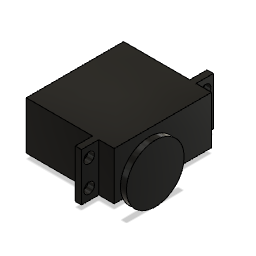
Servo Module v45 (Autodesk Fusion 360 archive; units mm, degrees)
design "HS-311"
Autodesk Fusion 360 part; units mm, degrees
sketch "Sketch1" plane through (0, 0, 0) normal (0, 0, 1) x (1, 0, 0) in component "MG995 v1 (1)"
  line L0 (-20.2, 9.95) -> (20.2, 9.95)
  line L1 (20.2, 9.95) -> (20.2, -9.95)
  line L2 (20.2, -9.95) -> (-20.2, -9.95)
  line L3 (-20.2, -9.95) -> (-20.2, 9.95)
  line L4 (0, 9.95) -> (0, -9.95) construction
  line L5 (-20.2, 0) -> (20.2, 0) construction
  dimension "d1_1_1_1_1" = 40.4
  dimension "d2_1_1_1_1" = 19.9
  constraint horizontal L0
  constraint vertical L1
  constraint horizontal L2
  constraint vertical L3
  constraint midpoint L0 L4.start
  constraint midpoint L2 L4.end
  constraint midpoint L3 L5.start
  constraint midpoint L1 L5.end
  constraint coincident origin L5
  constraint coincident origin L4
  measures "d1_1_1_1_1" distance of L0.start L0.end
  measures "d2_1_1_1_1" distance of L0.start L2.end
extrude "Extrude1" add sketch "Sketch1" along normal blind 36.5 in component "MG995 v1 (1)"
sketch "Sketch2" plane through (0, 0, 36.5) normal (0, 0, 1) x (1, 0, 0) in component "MG995 v1 (1)"
  line L0 (-20.2, -9.95) -> (20.2, -9.95)
  line L1 (20.2, -9.95) -> (20.2, 9.95)
  line L2 (20.2, 9.95) -> (-20.2, 9.95)
  line L3 (-20.2, 9.95) -> (-20.2, -9.95)
  line L4 (20.2, 9.95) -> (-20.2, 9.95)
  line L5 (-20.2, -9.95) -> (20.2, -9.95)
  line L6 (-10.7, 9.95) -> (-10.7, -9.95) construction
  circle A0 centre (-10.7, 0) radius 2.9
  line L7 (0, 9.95) -> (0, -9.95) construction
  dimension "d5_1_1_1_1" = 5.8
  dimension "d8_1_1_1_1" = 9.5
  constraint coincident L2 L6.start
  constraint coincident L0 L6.end
  constraint perpendicular L0 L6
  constraint midpoint L6 A0.centre
  constraint midpoint L4 L7.start
  constraint midpoint L5 L7.end
  measures "d5_1_1_1_1" diameter of A0
  measures "d8_1_1_1_1" distance of L3 L6
extrude "Extrude2" add sketch "Sketch2" along normal blind 5.06 contours A0 in component "MG995 v1 (1)"
ref_plane "WorkPlane1" through (0, 0, 27.5) normal (0, 0, -1) x (-1, 0, 0) in component "MG995 v1 (1)"
sketch "Sketch3" plane through (-4.1411, 18.8966, 27.5) normal (0, 0, -1) x (1, 0, 0) in component "MG995 v1 (1)"
  line L0 (31.5411, 8.9466) -> (-23.2589, 8.9466)
  line L1 (-23.2589, 8.9466) -> (-23.2589, 28.8466)
  line L2 (-23.2589, 28.8466) -> (31.5411, 28.8466)
  line L3 (31.5411, 28.8466) -> (31.5411, 8.9466)
  line L4 (24.3411, 28.8466) -> (-16.0589, 28.8466)
  line L5 (-16.0589, 8.9466) -> (24.3411, 8.9466)
  line L6 (24.3411, 8.9466) -> (24.3411, 28.8466)
  line L7 (-16.0589, 28.8466) -> (-16.0589, 8.9466)
  circle A0 centre (28.3411, 13.4466) radius 2.2
  circle A1 centre (28.3411, 24.3466) radius 2.2
  circle A2 centre (-20.0589, 13.4466) radius 2.2
  circle A3 centre (-20.0589, 24.3466) radius 2.2
  line L8 (28.3411, 8.9466) -> (28.3411, 28.8466) construction
  line L9 (-20.0589, 8.9466) -> (-20.0589, 28.8466) construction
  dimension "d10_1_1_1_1" = 7.2
  dimension "d11_1_1_1_1" = 7.2
  dimension "d12_1_1_1_1" = 4.4
  dimension "d13_1_1_1" = 4.4
  dimension "d14_1_1_1" = 4.4
  dimension "d15_1_1_1" = 4.4
  dimension "d16_1_1_1" = 4.5
  dimension "d17_1_1_1" = 4.5
  dimension "d18_1_1_1" = 4.5
  dimension "d19_1_1_1" = 4.5
  dimension "d20_1_1_1" = 3.2
  dimension "d21_1_1_1" = 3.2
  constraint horizontal L0
  constraint vertical L1
  constraint horizontal L2
  constraint vertical L3
  constraint collinear L2 L4
  constraint collinear L0 L5
  constraint coincident L0 L8.start
  constraint coincident L2 L8.end
  constraint perpendicular L2 L8
  constraint coincident L0 L9.start
  constraint coincident L2 L9.end
  constraint perpendicular L2 L9
  constraint coincident A0.centre L8
  constraint coincident A1.centre L8
  constraint coincident A2.centre L9
  constraint coincident A3.centre L9
  measures "d10_1_1_1_1" distance of L3 L6
  measures "d11_1_1_1_1" distance of L1 L7
  measures "d12_1_1_1_1" diameter of A0
  measures "d13_1_1_1" diameter of A1
  measures "d14_1_1_1" diameter of A2
  measures "d15_1_1_1" diameter of A3
  measures "d16_1_1_1" distance of L0 A0.centre
  measures "d17_1_1_1" distance of L2 A1.centre
  measures "d18_1_1_1" distance of L0 A2.centre
  measures "d19_1_1_1" distance of L2 A3.centre
  measures "d20_1_1_1" distance of L3 L8
  measures "d21_1_1_1" distance of L1 L9
extrude "Extrude3" add sketch "Sketch3" against normal blind 2.6 contours L0 L2 L3 L6 | L0 L1 L2 L7 in component "MG995 v1 (1)"
sketch "Sketch5" plane through (0, 0, 41.56) normal (0, 0, 1) x (1, 0, 0) in component "MG995 v1 (1)"
  circle A0 centre (-10.7, 0) radius 2.9
  circle A1 centre (-10.7, 0) radius 11.98
  dimension "d494_1_1_1" = 23.96
  constraint concentric A0 A1
  measures "d494_1_1_1" diameter of A1
extrude "Extrude5" add sketch "Sketch5" along normal blind 2.5 contours A0 | A1 in component "MG995 v1 (1)"
component "MG995 v1 (1)" placed x (0, 1, 0) y (0, 0, 1) z (1, 0, 0) at (-69.2471, 31.7306, -29.2908)
